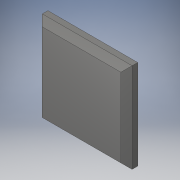
# Autodesk Inventor part: End Cap
Saved by Autodesk Inventor 2019 (Build 230136000, 136)
## iProperties
Created: 2018-11-11
Part Number: End Cap
Material: Generic
Document SubType Name: Modeling
Designer: maste
Density: 1 g/cm^3
Appearance: Default
Author: maste
Autodesk Inventor part; units mm, degrees
ref_plane "YZ Plane" through (0, 0, 0) normal (1, 0, 0) x (0, 1, 0)
ref_plane "XZ Plane" through (0, 0, 0) normal (0, 1, 0) x (-1, 0, 0)
ref_plane "XY Plane" through (0, 0, 0) normal (0, 0, 1) x (1, 0, 0)
sketch "Sketch1" plane through (0, 0, 0) normal (0, 0, 1) x (1, 0, 0)
  line L0 (0, 0) -> (50.8, 0)
  line L1 (50.8, 0) -> (50.8, 50.8)
  line L2 (50.8, 50.8) -> (0, 50.8)
  line L3 (0, 50.8) -> (0, 0)
  dimension "d0" = 50.8
  dimension "d1" = 50.8
  constraints: 8 end point, 2 parallel, 1 horizontal, 1 perpendicular
  measures "d0" distance of L2.end L1.end
  measures "d1" distance of L1.end L0.end
extrude "Extrusion1" add sketch "Sketch1" along normal blind 3.175
sketch "Sketch2" plane through (0, 0, 0) normal (0, 0, -1) x (-1, 0, 0)
  line L0 (0, 0) -> (-50.8, 0) projected
  line L1 (-50.8, 0) -> (-50.8, 50.8) projected
  line L2 (0, 0) -> (-50.8, 0)
  line L3 (-50.8, 0) -> (-50.8, 50.8)
  line L4 (-50.8, 50.8) -> (0, 50.8)
  line L5 (0, 50.8) -> (0, 0)
  line L6 (-3.175, 3.175) -> (-47.625, 3.175)
  line L7 (-47.625, 3.175) -> (-47.625, 47.625)
  line L8 (-47.625, 47.625) -> (-3.175, 47.625)
  line L9 (-3.175, 47.625) -> (-3.175, 3.175)
  dimension "d4" = 3.175
  constraints: 16 end point, 4 parallel, 2 perpendicular, 1 horizontal, 3 other
  measures "d4" distance between parallel lines of L5 L9
extrude "Extrusion2" add sketch "Sketch2" along normal blind 3.175 contours L6 L7 L8 L9
sketch "Sketch4" plane through (0, 0, 3.175) normal (0, 0, 1) x (1, 0, 0)
  line L0 (0, 0) -> (50.8, 0) projected
  line L1 (50.8, 0) -> (50.8, 50.8) projected
  line L2 (0, 0) -> (50.8, 0)
  line L3 (50.8, 0) -> (50.8, 50.8)
  line L4 (50.8, 50.8) -> (0, 50.8)
  line L5 (0, 50.8) -> (0, 0)
  constraints: 8 end point, 2 parallel, 1 horizontal, 1 perpendicular
extrude "Extrusion4" add sketch "Sketch4" along normal blind 3.175
chamfer "Chamfer1" distance 3.175 angle 45 4 edges at (50.8, 25.4, 6.35) (25.4, 0, 6.35) (0, 25.4, 6.35) (25.4, 50.8, 6.35)
body "Solid1"
